Autodesk Fusion 360 part; units mm, degrees
(part 2 of 2)
  constraint concentric A1 A249
  constraint concentric A4 A251
  constraint concentric A251 A255
  constraint concentric A3 A252
  constraint concentric A252 A253
  constraint coincident L181.end A253
  constraint concentric A253 A254
  constraint coincident L189.end A255
  constraint concentric A255 A256
  constraint coincident L134.end A257
  constraint concentric A257 A258
  measures "d1" diameter of A0
  measures "d2" diameter of A1
  measures "d3" diameter of A2
  measures "d4" diameter of A3
  measures "d5" diameter of A4
  measures "d9" diameter of A111
  measures "d12" diameter of A112
  measures "d255" diameter of A249
  measures "d256" diameter of A250
  measures "d257" diameter of A251
  measures "d259" diameter of A252
extrude "Extrude1" add sketch "mriya" along normal blind 10.5 contours L201 A203 L202 A204 L203 A205 L204 A206 L205 A207 L206 A208 L207 A209 L208 A210 L209 A211 L210 A212 L211 A213 L212 A214 L213 A215 L214 A216 L215 L216 A218 L217 A219 L218 A220 L219 A221 L220 A222 L221 A223 L222 A224 L223 L224 L225 A225 L226 A226 L227 L228 L229 L230 L231 L232 L233 L234 L235 L236 L237 L238 A228 L239 L240 L241 L242 L243 L244 A229 A230 A231 A232 A233 A234 A235 A236 L245 A237 A238 A239 A240 A241 A242 A243 A244 A245 A246 L248 makes body 1
extrude "Extrude2" add sketch "mriya" along normal blind 17 contours L215 A217 L216 L237 A227 L238 L245 L248 bodies 1
extrude "Extrude3" add sketch "mriya" along normal blind 3.7 contours L106 L107 L108 A113 A114 A115 L109 L110 A116 A117 L201 A203 L202 A204 L203 A205 L204 A206 L205 A207 L206 A208 L207 A209 L208 A210 L209 A211 L210 A212 L211 A213 L212 A214 L213 A215 L214 A216 L215 L216 A218 L217 A219 L218 A220 L219 A221 L220 A222 L221 A223 L222 A224 L246 L247 | L106 L107 L108 A113 A114 A115 L215 A217 L216 L246 | L109 L110 A116 A117 L215 L247 | A119 | A120 | A121 | A122 bodies 1
extrude "Extrude6" add sketch "mriya" along normal blind 1 from surface at 14.3 contours L106 L107 L108 A113 A114 A115 L215 A217 L216 L246 bodies 1
extrude "Extrude7" add sketch "mriya" along normal blind 1 from surface at 7.8 contours L109 L110 A116 A117 L215 L247 bodies 1
sketch "power-switch" plane through (-4.45, 0, 0) normal (1, 0, 0) x (0, 1, 0)
  line L0 (19.1932, 0) -> (76.4932, 0)
  line L1 (76.4932, 0) -> (76.4932, 16.8)
  line L2 (76.4932, 16.8) -> (19.1932, 16.8)
  line L3 (19.1932, 16.8) -> (19.1932, 10.5)
  line L4 (36.0932, 5.1) -> (25.6932, 5.1)
  line L5 (25.6932, 5.1) -> (25.6932, 8)
  line L6 (25.6932, 8) -> (36.0932, 8)
  line L7 (36.0932, 8) -> (36.0932, 5.1)
  line L8 (37.1932, 3.25) -> (24.5932, 3.25)
  line L9 (23.5932, 4.25) -> (23.5932, 8.85)
  line L10 (24.5932, 9.85) -> (37.1932, 9.85)
  line L11 (38.1932, 8.85) -> (38.1932, 4.25)
  arc A0 (24.5932, 9.85) -> (23.5932, 8.85) centre (24.5932, 8.85) ccw
  arc A1 (38.1932, 8.85) -> (37.1932, 9.85) centre (37.1932, 8.85) ccw
  arc A2 (37.1932, 3.25) -> (38.1932, 4.25) centre (37.1932, 4.25) ccw
  arc A3 (23.5932, 4.25) -> (24.5932, 3.25) centre (24.5932, 4.25) ccw
  line L12 (19.1932, 10.5) -> (19.1932, 0)
  line L13 (1.9932, 0) -> (76.4932, 0)
  line L14 (76.4932, 0) -> (76.4932, 17)
  line L15 (76.4932, 17) -> (19.1932, 17)
  line L16 (19.1932, 17) -> (19.1932, 10.5)
  line L17 (19.1932, 10.5) -> (1.9932, 10.5)
  line L18 (1.9932, 10.5) -> (1.9932, 0)
  constraint perpendicular L4 L5
  constraint tangent L9 A0
  constraint tangent L10 A0
  constraint tangent L10 A1
  constraint tangent L11 A1
  constraint tangent L8 A2
  constraint tangent L11 A2
  constraint tangent L8 A3
  constraint tangent L9 A3
  constraint vertical L5
  constraint perpendicular L5 L6
  constraint vertical L7
extrude "Extrude8" cut sketch "power-switch" against normal blind 2.5 contours L4 L5 L6 L7 bodies 1
extrude "Extrude9" cut sketch "power-switch" against normal blind 1.2 contours L8 L9 L10 L11 A0 A1 A2 A3 bodies 1
chamfer "Chamfer5" distance 0.5 angle 45 4 edges at (-6.95, 30.8932, 5.1) (-6.95, 36.0932, 6.55) (-6.95, 30.8932, 8) (-6.95, 25.6932, 6.55) on bodies 1
sketch "usb-c" plane through (0, 80.6432, 0) normal (0, 1, 0) x (-1, 0, 0)
  line L0 (3.6, 0) -> (36.1295, 0)
  line L1 (3.6, 16.7) -> (3.6, 0)
  line L2 (21.2003, 10.9) -> (21.2003, 10.1)
  arc A0 (21.2003, 10.9) -> (19.8003, 12.3) centre (19.8003, 10.9) ccw
  line L3 (11.8003, 10.1) -> (11.8003, 10.9)
  line L4 (19.8003, 8.7) -> (13.2003, 8.7)
  line L5 (21.5003, 7) -> (11.5002, 7)
  arc A1 (11.8003, 10.1) -> (13.2003, 8.7) centre (13.2003, 10.1) ccw
  line L6 (22.7003, 12.8) -> (22.7003, 8.2)
  line L7 (11.5003, 14) -> (21.5003, 14)
  arc A2 (13.2002, 12.3) -> (11.8002, 10.9) centre (13.2002, 10.9) ccw
  arc A3 (19.8003, 8.7) -> (21.2003, 10.1) centre (19.8003, 10.1) ccw
  line L8 (10.3003, 8.2) -> (10.3003, 12.8)
  line L9 (13.2002, 12.3) -> (19.8003, 12.3)
  line L10 (8.6, 0) -> (25.9, 0)
  line L11 (25.9, 10.5) -> (25.9, 16.8)
  line L12 (25.9, 16.8) -> (8.6, 16.8)
  line L13 (8.6, 16.8) -> (8.6, 0)
  arc A4 (22.7003, 12.8) -> (21.5003, 14) centre (21.5003, 12.8) ccw
  arc A5 (21.5003, 7) -> (22.7002, 8.2) centre (21.5002, 8.2) ccw
  arc A6 (10.3003, 8.2) -> (11.5002, 7) centre (11.5003, 8.2) ccw
  arc A7 (11.5003, 14) -> (10.3003, 12.8) centre (11.5003, 12.8) ccw
  line L14 (25.9, 0) -> (25.9, 10.5)
  line L15 (8.6, 0) -> (41.0881, 0)
  line L16 (41.0881, 0) -> (41.0881, 10.5)
  line L17 (41.0881, 10.5) -> (25.9, 10.5)
  line L18 (25.9, 10.5) -> (25.9, 17)
  line L19 (25.9, 17) -> (8.6, 17)
  line L20 (8.6, 17) -> (8.6, 0)
  line L21 (21.2003, 10.5) -> (21.5857, 10.5)
  constraint tangent L3 A2
  constraint tangent A2 L9
  constraint tangent A0 L9
  constraint tangent L2 A0
  constraint tangent L4 A3
  constraint tangent L2 A3
  constraint tangent L4 A1
  constraint tangent L3 A1
  constraint perpendicular L6 L7
  constraint perpendicular L5 L8
  constraint horizontal L5
  constraint perpendicular L5 L6
  constraint tangent L7 A4
  constraint tangent L6 A4
  constraint tangent L6 A5
  constraint tangent L5 A5
  constraint tangent L5 A6
  constraint tangent L8 A6
  constraint tangent L7 A7
  constraint tangent L8 A7
  constraint midpoint L2 L21.start
  constraint perpendicular L2 L21
extrude "Extrude10" cut sketch "usb-c" against normal blind 2.5 contours L2 A0 L3 L4 A1 A2 A3 L9 bodies 1
extrude "Extrude11" cut sketch "usb-c" against normal blind 1.2 contours L5 L6 L7 L8 A4 A5 A6 A7 bodies 1
chamfer "Chamfer3" distance 0.9 angle 45 4 edges at (-6.95, 9.5932, 7.8) (-6.95, 48.8432, 14.3) (-7.4333, 77.6599, 14.3) (-16.65, 78.1432, 14.3) on bodies 1
chamfer "Chamfer4" distance 1 angle 45 90 edges at (-33.4941, 80.6432, 10.5) (-41.4708, 80.7193, 10.5) (-42.3594, 81.5003, 10.5) (-43.8969, 82.7148, 10.5) (-51.4665, 82.9432, 10.5) (-58.2721, 83.0196, 10.5) (-60.2606, 84.9007, 10.5) (-62.897, 87.2147, 10.5) (-73.4001, 87.4432, 10.5) (-83.9031, 87.2148, 10.5) (-86.0406, 85.4003, 10.5) (-87.5292, 84.0193, 10.5) (-94.8335, 83.9432, 10.5) (-102.9031, 83.7148, 10.5) (-107.2173, 79.7235, 10.5) (-111.045, 76.0574, 10.5) (-116.187, 75.9432, 10.5) (-121.9031, 75.7148, 10.5) (-123.4406, 74.5003, 10.5) (-124.3292, 73.7193, 10.5) (-131.4059, 73.6432, 10.5) (-141.0345, 72.4277, 10.5) (-142.25, 42.8932, 10.5) (-141.0345, 13.3587, 10.5) (-120.383, 12.1432, 10.5) (-100.9441, 12.4856, 10.5) (-96.4346, 16.5099, 10.5) (-92.7374, 19.9914, 10.5) (-84.5856, 20.1432, 10.5) (-75.6851, 19.7342, 10.5) (-70.5182, 11.4202, 10.5) (-65.1681, 2.9203, 10.5) (-56.0579, 2.4432, 10.5) (-48.3292, 2.3671, 10.5) (-47.4406, 1.5861, 10.5) (-45.9031, 0.3716, 10.5) (-37.2335, 0.1432, 10.5) (-29.3403, 0.0695, 10.5) (-28.4501, -0.712, 10.5) (-26.9041, -1.93, 10.5) (-17.1798, -2.1568, 10.5) (-5.6655, -0.9413, 10.5) (-4.45, 10.5932, 10.5) (-17.25, 80.6432, 17) (-4.45, 47.8432, 17) (-5.6655, 79.4277, 17) (-4.45, 39.2432, 0) (-5.6655, 79.4277, 0) (-24.8441, 80.6432, 0) (-41.4708, 80.7193, 0) (-42.3594, 81.5003, 0) (-43.8969, 82.7148, 0) (-51.4665, 82.9432, 0) (-58.2721, 83.0196, 0) (-60.2606, 84.9007, 0) (-62.897, 87.2147, 0) (-73.4001, 87.4432, 0) (-83.9031, 87.2148, 0) (-86.0406, 85.4003, 0) (-87.5292, 84.0193, 0) (-94.8335, 83.9432, 0) (-102.9031, 83.7148, 0) (-107.2173, 79.7235, 0) (-111.045, 76.0574, 0) (-116.187, 75.9432, 0) (-121.9031, 75.7148, 0) (-123.4406, 74.5003, 0) (-124.3292, 73.7193, 0) (-131.4059, 73.6432, 0) (-141.0345, 72.4277, 0) (-142.25, 42.8932, 0) (-141.0345, 13.3587, 0) (-120.383, 12.1432, 0) (-100.9441, 12.4856, 0) (-96.4346, 16.5099, 0) (-92.7374, 19.9914, 0) (-84.5856, 20.1432, 0) (-75.6851, 19.7342, 0) (-70.5182, 11.4202, 0) (-65.1681, 2.9203, 0) (-56.0579, 2.4432, 0) (-48.3292, 2.3671, 0) (-47.4406, 1.5861, 0) (-45.9031, 0.3716, 0) (-37.2335, 0.1432, 0) (-29.3403, 0.0695, 0) (-28.4501, -0.712, 0) (-26.9041, -1.93, 0) (-17.1798, -2.1568, 0) (-5.6655, -0.9413, 0) on bodies 1
fillet "Fillet27" radius 1.2 1 edges at (-4.45, 19.1932, 12.75) on bodies 1
chamfer "Chamfer6" distance 1 angle 45 2 edges at (-6.3, 19.1932, 17) (-5.5496, 19.1974, 17) on bodies 1
extrude "Extrude12" add sketch "mriya" along normal blind 1.7 contours A2 | L113 L114 L115 L116 A123 A124 A125 A247 | L117 A126 L118 A127 L119 A128 L120 A257 | A129 L121 A130 L122 A131 L123 A132 L124 | A133 L125 A134 L126 A135 L127 A136 L128 | A137 L129 A138 L130 L131 A139 L132 A248 | A140 L133 A141 L134 L135 A142 L136 A258 | A143 L137 A144 L138 A145 L139 A146 L140 | A147 L141 A148 L142 A149 L143 A150 L144 | A151 L145 A152 L146 A153 L147 A154 L148 | A155 L149 A156 L150 A157 L151 A158 L152 | A159 L153 A160 L154 A161 L155 A162 L156 | A163 L157 A164 L158 A165 L159 A166 L160 | A167 L161 A168 L162 A169 L163 A170 L164 | A171 L165 A172 L166 A173 L167 L168 A255 | A174 L169 A175 L170 A176 L171 A177 L172 | A178 L173 A179 L174 A180 L175 L176 A253 | A181 L177 A182 L178 A183 L179 A184 L180 | A185 L181 L182 A186 L183 A187 L184 A254 | A188 L185 A189 L186 A190 L187 A191 L188 | A192 L189 L190 A193 L191 A194 L192 A256 | A195 L193 A196 L194 A197 L195 A198 L196 | A199 L197 A200 L198 A201 L199 A202 L200 bodies 1
sketch "bottom" plane through (0, 0, 0) normal (0, 0, -1) x (1, 0, 0)
  circle A0 centre (-44.9, -22.5432) radius 1.6
  circle A1 centre (-120.9, -34.5432) radius 1.6
  circle A2 centre (-120.9, -53.5432) radius 1.6
  circle A3 centre (-44.9, -60.5432) radius 1.6
  line L0 (-5.45, -76.4932) -> (-5.45, -1.9932)
  arc A4 (-5.45, -1.9932) -> (-8.6, 1.1568) centre (-8.6, -1.9932) ccw
  line L1 (-8.6, 1.1568) -> (-25.7597, 1.1568)
  arc A5 (-25.7597, 1.1568) -> (-27.1701, 0.5748) centre (-25.7597, -0.8432) ccw
  line L2 (-27.1701, 0.5748) -> (-28.3196, -0.5687)
  arc A6 (-29.7119, -1.1432) -> (-28.3196, -0.5687) centre (-29.7119, 0.831) ccw
  line L3 (-29.7119, -1.1432) -> (-44.755, -1.1432)
  arc A7 (-44.755, -1.1432) -> (-46.1692, -1.729) centre (-44.755, -3.1432) ccw
  line L4 (-46.1692, -1.729) -> (-47.2977, -2.8574)
  arc A8 (-48.7119, -3.4432) -> (-47.2977, -2.8574) centre (-48.7119, -1.4432) ccw
  line L5 (-48.7119, -3.4432) -> (-63.4039, -3.4432)
  arc A9 (-63.4039, -3.4432) -> (-65.5806, -4.7135) centre (-63.4039, -5.9432) ccw
  line L6 (-65.5806, -4.7135) -> (-73.7146, -19.1108)
  arc A10 (-77.1972, -21.1432) -> (-73.7146, -19.1108) centre (-77.1972, -17.1432) ccw
  line L7 (-77.1972, -21.1432) -> (-91.9739, -21.1432)
  arc A11 (-94.0918, -20.2661) -> (-91.9739, -21.1432) centre (-91.9739, -18.1477) ccw
  line L8 (-94.0918, -20.2661) -> (-100.1914, -14.168)
  arc A12 (-100.1914, -14.168) -> (-102.666, -13.1432) centre (-102.666, -16.6432) ccw
  line L9 (-102.666, -13.1432) -> (-138.1, -13.1432)
  arc A13 (-138.1, -13.1432) -> (-141.25, -16.2932) centre (-138.1, -16.2932) ccw
  line L10 (-141.25, -16.2932) -> (-141.25, -69.4932)
  arc A14 (-141.25, -69.4932) -> (-138.1, -72.6432) centre (-138.1, -69.4932) ccw
  line L11 (-138.1, -72.6432) -> (-124.7119, -72.6432)
  arc A15 (-123.2977, -73.229) -> (-124.7119, -72.6432) centre (-124.7119, -74.6432) ccw
  line L12 (-123.2977, -73.229) -> (-122.1692, -74.3574)
  arc A16 (-122.1692, -74.3574) -> (-120.755, -74.9432) centre (-120.755, -72.9432) ccw
  line L13 (-120.755, -74.9432) -> (-111.619, -74.9432)
  arc A17 (-109.8512, -75.6754) -> (-111.619, -74.9432) centre (-111.619, -77.4432) ccw
  line L14 (-109.8512, -75.6754) -> (-103.1692, -82.3574)
  arc A18 (-103.1692, -82.3574) -> (-101.755, -82.9432) centre (-101.755, -80.9432) ccw
  line L15 (-101.755, -82.9432) -> (-87.9119, -82.9432)
  arc A19 (-86.4977, -83.529) -> (-87.9119, -82.9432) centre (-87.9119, -84.9432) ccw
  line L16 (-86.4977, -83.529) -> (-84.1692, -85.8574)
  arc A20 (-84.1692, -85.8574) -> (-82.755, -86.4432) centre (-82.755, -84.4432) ccw
  line L17 (-82.755, -86.4432) -> (-64.0453, -86.4432)
  arc A21 (-64.0453, -86.4432) -> (-62.6308, -85.8572) centre (-64.0453, -84.4432) ccw
  line L18 (-62.6308, -85.8572) -> (-59.3049, -82.5302)
  arc A22 (-57.8881, -81.9432) -> (-59.3049, -82.5302) centre (-57.8881, -83.9465) ccw
  line L19 (-57.8881, -81.9432) -> (-45.045, -81.9432)
  arc A23 (-45.045, -81.9432) -> (-43.6308, -81.3574) centre (-45.045, -79.9432) ccw
  line L20 (-43.6308, -81.3574) -> (-42.5023, -80.229)
  arc A24 (-41.0881, -79.6432) -> (-42.5023, -80.229) centre (-41.0881, -81.6432) ccw
  line L21 (-41.0881, -79.6432) -> (-8.6, -79.6432)
  arc A25 (-8.6, -79.6432) -> (-5.45, -76.4932) centre (-8.6, -76.4932) ccw
  circle A26 centre (-44.9, -60.5432) radius 2
  circle A27 centre (-44.9, -22.5432) radius 2
  circle A28 centre (-120.9, -53.5432) radius 2
  circle A29 centre (-120.9, -34.5432) radius 2
  circle A30 centre (-10.95, -74.1432) radius 4
  circle A31 centre (-10.95, -4.3432) radius 4
  circle A32 centre (-61.6532, -8.9432) radius 4
  circle A33 centre (-73.4001, -80.9432) radius 4
  circle A34 centre (-135.75, -67.1432) radius 4
  circle A35 centre (-135.75, -18.6432) radius 4
  dimension "d261" = 4
  dimension "d262" = 4
  dimension "d263" = 4
  dimension "d264" = 4
  dimension "d265" = 8
  dimension "d266" = 8
  dimension "d267" = 8
  dimension "d268" = 8
  dimension "d269" = 8
  dimension "d270" = 8
  dimension "d271" = 5.5
  dimension "d272" = 5.5
  dimension "d273" = 5.5
  dimension "d274" = 5.5
  dimension "d275" = 5.5
  dimension "d276" = 5.5
  dimension "d277" = 5.5
  dimension "d278" = 5.5
  dimension "d279" = 5.5
  dimension "d280" = 5.5
  dimension "d281" = 5.5
  constraint concentric A3 A26
  constraint concentric A0 A27
  constraint concentric A2 A28
  constraint concentric A1 A29
  measures "d261" diameter of A26
  measures "d262" diameter of A27
  measures "d263" diameter of A28
  measures "d264" diameter of A29
  measures "d265" diameter of A30
  measures "d266" diameter of A31
  measures "d267" diameter of A32
  measures "d268" diameter of A33
  measures "d269" diameter of A34
  measures "d270" diameter of A35
  measures "d271" distance of L0 A30.centre
  measures "d272" distance of L21 A30.centre
  measures "d273" distance of L1 A31.centre
  measures "d274" distance of L0 A31.centre
  measures "d275" distance of L6 A32.centre
  measures "d276" distance of L5 A32.centre
  measures "d277" distance of L10 A35.centre
  measures "d278" distance of L9 A35.centre
  measures "d279" distance of L10 A34.centre
  measures "d280" distance of L11 A34.centre
  measures "d281" distance of L17 A33.centre
extrude "Extrude13" add sketch "mriya" along normal blind 1.7 contours A0 | A1 | A3 | A4 bodies 1
extrude "Extrude14" cut sketch "bottom" against normal blind 0.8 contours A0 | A1 | A2 | A3 | A26 | A27 | A28 | A29 | A30 | A31 | A32 | A33 | A34 | A35 bodies 1
chamfer "Chamfer7" distance 0.7 angle 45 8 edges at (-4.45, 38.1932, 6.55) (-4.45, 37.9003, 3.5429) (-4.45, 30.8932, 3.25) (-4.45, 23.8861, 3.5429) (-4.45, 23.5932, 6.55) (-4.45, 23.8861, 9.5571) (-4.45, 30.8932, 9.85) (-4.45, 37.9003, 9.5571) on bodies 1
chamfer "Chamfer8" distance 0.7 angle 45 8 edges at (-22.7003, 80.6432, 10.5) (-22.3488, 80.6432, 7.3515) (-16.5002, 80.6432, 7) (-10.6517, 80.6432, 7.3515) (-10.3003, 80.6432, 10.5) (-10.6517, 80.6432, 13.6485) (-16.5003, 80.6432, 14) (-22.3488, 80.6432, 13.6485) on bodies 1
mirror "Mirror1" about plane through (0, 0, 0) normal (1, 0, 0) of bodies 1 makes body 2
named bodies: "Left", "Right"
